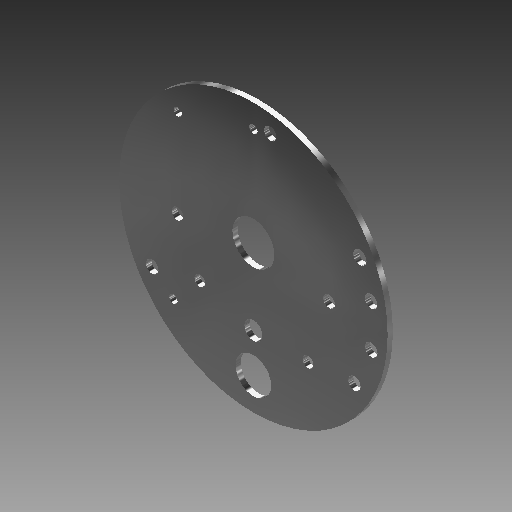
# Autodesk Inventor part: 403-01
Saved by Autodesk Inventor 2019 (Build 230136000, 136)
## iProperties
Company: Autodesk Inc.
Created: 2017-06-27
Part Number: 403-01
Material: Aluminum-6061
Document SubType Name: Modeling
Designer: Autodesk Inc.
Mass: 10.0284 g
Surface Area: 64.2025 cm^2
Volume: 3.71421 cm^3
Density: 2.7 g/cm^3
Appearance: Chrome - Polished
Author: Inventor
Autodesk Inventor part; units mm, degrees
ref_plane "YZ Plane" through (0, 0, 0) normal (1, 0, 0) x (0, 1, 0)
ref_plane "XZ Plane" through (0, 0, 0) normal (0, 1, 0) x (-1, 0, 0)
ref_plane "XY Plane" through (0, 0, 0) normal (0, 0, 1) x (1, 0, 0)
sketch "Sketch1" plane through (0, 0, 0) normal (0, 0, 1) x (1, 0, 0)
  circle A0 centre (0, 0) radius 31.9
  dimension "d0" = 63.8
  constraints: 1 centre point, 1 coincident
  measures "d0" diameter of A0
extrude "Extrusion1" add sketch "Sketch1" against normal blind 1.25
sketch "Sketch2" plane through (0, 0, 0) normal (0, 0, 1) x (1, 0, 0)
  point P0 (0, 0)
  point P1 (-19, -18)
  dimension "d3" = 19
  dimension "d4" = 18
  measures "d3" horizontal distance of point (0, 0) point (-19, -18)
  measures "d4" vertical distance of point (0, 0) point (-19, -18)
hole "Hole1" at (-19, -18, 0) direction (0, 0, -1) diameter 2 end through all
sketch "Sketch3" plane through (0, 0, 0) normal (0, 0, 1) x (1, 0, 0)
  point P0 (0, 0)
  point P1 (-17.9556, 21)
  point P2 (0, 26.4)
  dimension "d12" = 26.4
  dimension "d101" = 18.75
  dimension "d102" = 21
  constraints: 1 vertical alignment
  measures "d12" distance of point (0, 26.4) point (0, 0)
  measures "d101" distance of point (0, 26.4) point (-17.956, 21)
  measures "d102" vertical distance of point (0, 0) point (-17.956, 21)
hole "Hole2" at (-17.9556, 21, 0) at (0, 26.4, 0) direction (0, 0, -1) diameter 2 end through all
sketch "Sketch4" plane through (0, 0, 0) normal (0, 0, 1) x (1, 0, 0)
  point P0 (0, 0)
  point P1 (-12.7, -11.1)
  point P2 (13, -15)
  dimension "d22" = 15
  dimension "d23" = 11.1
  dimension "d24" = 12.7
  dimension "d25" = 13
  measures "d22" vertical distance of point (13, -15) point (0, 0)
  measures "d23" vertical distance of point (-12.7, -11.1) point (0, 0)
  measures "d24" horizontal distance of point (0, 0) point (-12.7, -11.1)
  measures "d25" horizontal distance of point (0, 0) point (13, -15)
hole "Hole3" at (-12.7, -11.1, 0) at (13, -15, 0) direction (0, 0, -1) diameter 2.6 end through all
sketch "Sketch5" plane through (0, 0, 0) normal (0, 0, 1) x (1, 0, 0)
  line L0 (-18, 0) -> (18, 0) construction
  point P0 (0, 0)
  point P1 (0, 0)
  dimension "d33" = 36
  constraints: 2 end point, 1 coincident, 1 horizontal, 1 midpoint
  measures "d33" distance of L0.start L0.end
hole "Hole4" at (18, 0, 0) at (-18, 0, 0) direction (0, 0, -1) diameter 2.8 end through all
sketch "Sketch6" plane through (0, 0, 0) normal (0, 0, 1) x (1, 0, 0)
  point P0 (0, 0)
  point P1 (24, -13.9)
  point P2 (-24, -13.9)
  point P3 (4, 27.5)
  dimension "d41" = 24
  dimension "d42" = 13.9
  dimension "d59" = 4
  dimension "d61" = 24
  dimension "d62" = 13.9
  dimension "d63" = 27.5
  measures "d41" horizontal distance of point (24, -13.9) point (0, 0)
  measures "d42" vertical distance of point (0, 0) point (24, -13.9)
  measures "d59" horizontal distance of point (4, 27.5) point (0, 0)
  measures "d61" horizontal distance of point (0, 0) point (-24, -13.9)
  measures "d62" vertical distance of point (-24, -13.9) point (0, 0)
  measures "d63" vertical distance of point (0, 0) point (4, 27.5)
hole "Hole5" at (24, -13.9, 0) at (4, 27.5, 0) at (-24, -13.9, 0) direction (0, 0, -1) diameter 3 end through all
sketch "Sketch7" plane through (0, 0, 0) normal (0, 0, 1) x (1, 0, 0)
  point P0 (0, 0)
  point P1 (25.3, 12.7)
  dimension "d50" = 12.7
  dimension "d51" = 25.3
  measures "d50" vertical distance of point (25.3, 12.7) point (0, 0)
  measures "d51" horizontal distance of point (25.3, 12.7) point (0, 0)
hole "Hole6" at (25.3, 12.7, 0) direction (0, 0, -1) diameter 3.2 end through all
sketch "Sketch8" plane through (0, 0, 0) normal (0, 0, 1) x (1, 0, 0)
  point P0 (0, 0)
  point P1 (0, -15)
  dimension "d64" = 15
  constraints: 1 vertical alignment
  measures "d64" distance of point (0, -15) point (0, 0)
hole "Hole7" at (0, -15, 0) direction (0, 0, -1) diameter 4.3 end through all
sketch "Sketch10" plane through (0, 0, 0) normal (0, 0, 1) x (1, 0, 0)
  point P0 (0, 0)
  point P1 (0, 3)
  dimension "d81" = 3
  constraints: 1 vertical alignment
  measures "d81" distance of point (0, 3) point (0, 0)
hole "Hole9" at (0, 3, 0) direction (0, 0, -1) diameter 10 end through all
sketch "Sketch11" plane through (0, 0, 0) normal (0, 0, 1) x (1, 0, 0)
  point P0 (0, 0)
  point P1 (0, 0)
  point P2 (28, -5)
  point P3 (28, 5)
  dimension "d91" = 28
  dimension "d92" = 5
  dimension "d93" = 5
  constraints: 1 vertical alignment
  measures "d91" horizontal distance of point (28, -5) point (0, 0)
  measures "d92" vertical distance of point (0, 0) point (28, -5)
  measures "d93" vertical distance of point (28, 5) point (0, 0)
hole "Hole10" at (28, -5, 0) at (28, 5, 0) direction (0, 0, -1) diameter 3 end through all
sketch "Sketch12" plane through (0, 0, -1.25) normal (0, 0, -1) x (-1, 0, 0)
  circle A0 centre (0, 0) radius 31.875
  line L0 (0, 0) -> (0, -24.3) construction
  circle A1 centre (0, -24.3) radius 4.25
  point P0 (-3.6509, -26.4756)
  point P1 (3.6509, -26.4756)
  point P2 (-3.6509, -22.1244)
  point P3 (3.6509, -22.1244)
  dimension "d103" = 24.3
  dimension "d104" = 8.5
  dimension "d105" = 63.75
  constraints: 4 point on circle, 2 centre point, 2 end point, 1 coincident
  measures "d103" distance of L0.start L0.end
  measures "d104" diameter of A1
  measures "d105" diameter of A0
extrude "Extrusion2" cut sketch "Sketch12" against normal through all contours A1
equation "\"d62\" = d42"
equation "\"d93\" = d92"
body "Solid1"
